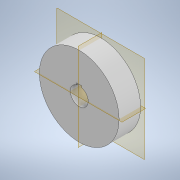
# Autodesk Inventor part: gear4
Saved by Autodesk Inventor 2022 (Build 260153000, 153)
## iProperties
Created: 2023-12-21
Part Number: gear4
Material: 一般
Document SubType Name: Modeling
Designer: ktamu
Density: 1 g/cm^3
Appearance: 既定
Author: ktamu
Autodesk Inventor part; units mm, degrees
sketch "スケッチ1" plane through (0, 0, 0) normal (0, 0, 1) x (1, 0, 0)
  circle A0 centre (0, 0) radius 111
  arc A1 (-7, 24) -> (7, 24) centre (0, 0) ccw
  line L0 (0, 25) -> (0, 28.8)
  line L1 (0, 28.8) -> (0, 20)
  line L2 (0, 20) -> (-7, 20)
  line L3 (-7, 24) -> (-7, 28.8)
  line L4 (-7, 28.8) -> (7, 28.8)
  line L5 (7, 28.8) -> (7, 24)
  line L6 (7, 20) -> (0, 20)
  dimension "d0" = 222
  dimension "d1" = 50
  dimension "d2" = 3.8
  dimension "d3" = 8.8
  dimension "d4" = 7
  dimension "d5" = 14
  constraints: 14 end point, 5 perpendicular, 3 point on line, 2 centre point, 2 coincident, 2 point on circle, 1 vertical
  measures "d0" diameter of A0
  measures "d1" diameter of A1
  measures "d2" distance of L0.start L0.end
  measures "d3" distance of L0.end L1.end
  measures "d4" distance of L1.end L2.end
  measures "d5" distance of L3.end L4.end
extrude "押し出し1" add sketch "スケッチ1" along normal blind 60
